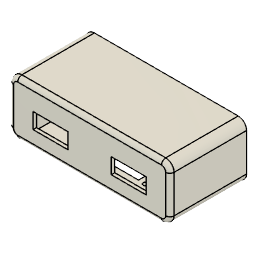
Qbot Head (Autodesk Fusion 360 design; units mm, degrees)
part number: 2026-07-07-13-50-28-448
Autodesk Fusion 360 part; units mm, degrees
sketch "Sketch1" plane through (0, 0, 0) normal (0, 0, 1) x (1, 0, 0)
  line L0 (0, 0) -> (-115, 0)
  line L1 (-115, 0) -> (-115, 39)
  line L2 (-115, 39) -> (0, 39)
  line L3 (0, 39) -> (0, 0)
  circle A0 centre (-5, 34) radius 2.6
  circle A1 centre (-5, 34) radius 1.6
  circle A2 centre (-5, 5) radius 2.6
  circle A3 centre (-5, 5) radius 1.6
  circle A4 centre (-110, 5) radius 2.6
  circle A5 centre (-110, 5) radius 1.6
  circle A6 centre (-110, 34) radius 2.6
  circle A7 centre (-110, 34) radius 1.6
  line L4 (-10, 35.5) -> (-105, 35.5)
  line L5 (-105, 35.5) -> (-105, 3.5)
  line L6 (-105, 3.5) -> (-10, 3.5)
  line L7 (-10, 3.5) -> (-10, 35.5)
  dimension "d1" = 115
  dimension "d2" = 39
  dimension "d3" = 5.2
  dimension "d4" = 5
  dimension "d5" = 5
  dimension "d6" = 3.2
  dimension "d7" = 5.2
  dimension "d8" = 5
  dimension "d9" = 5
  dimension "d10" = 3.2
  dimension "d11" = 5.2
  dimension "d12" = 5
  dimension "d13" = 5
  dimension "d14" = 3.2
  dimension "d15" = 5.2
  dimension "d16" = 5
  dimension "d17" = 5
  dimension "d18" = 3.2
  dimension "d19" = 95
  dimension "d20" = 32
  dimension "d21" = 10
  dimension "d22" = 3.5
  constraint horizontal L0
  constraint vertical L1
  constraint horizontal L2
  constraint vertical L3
  constraint coincident L0.start L3.end
  constraint concentric A0 A1
  constraint concentric A2 A3
  constraint concentric A4 A5
  constraint concentric A6 A7
  constraint horizontal L4
  constraint vertical L5
  constraint horizontal L6
  constraint vertical L7
  measures "d1" distance of L0.start L0.end
  measures "d2" distance of L0.start L2.end
  measures "d3" diameter of A0
  measures "d4" distance of L2 A0.centre
  measures "d5" distance of L3 A0.centre
  measures "d6" diameter of A1
  measures "d7" diameter of A2
  measures "d8" distance of L0 A2.centre
  measures "d9" distance of L3 A2.centre
  measures "d10" diameter of A3
  measures "d11" diameter of A4
  measures "d12" distance of L0 A4.centre
  measures "d13" distance of L1 A4.centre
  measures "d14" diameter of A5
  measures "d15" diameter of A6
  measures "d16" distance of L1 A6.centre
  measures "d17" distance of L2 A6.centre
  measures "d18" diameter of A7
  measures "d19" distance of L4.start L4.end
  measures "d20" distance of L4.start L6.end
  measures "d21" distance of L3 L7
  measures "d22" distance of L0 L6
extrude "Extrude1" add sketch "Sketch1" along normal blind 55 contours L0 L1 L2 L3 | A0 | A1 | A2 | A3 | A4 | A5 | A6 | A7 | L4 L5 L6 L7
extrude "Extrude2" cut sketch "Sketch1" along normal blind 52.5 contours L4 L5 L6 L7
extrude "Extrude3" cut sketch "Sketch1" along normal blind 5 contours A0 | A2 | A4 | A6
extrude "Extrude4" cut sketch "Sketch1" along normal blind 15 contours A1 | A3 | A5 | A7
sketch "Sketch2" plane through (0, 0, 0) normal (0, 1, 0) x (1, 0, 0)
  line L0 (-27.5, -10) -> (-82.5, -10)
  line L1 (-82.5, -10) -> (-82.5, -45)
  line L2 (-82.5, -45) -> (-27.5, -45)
  line L3 (-27.5, -45) -> (-27.5, -10)
  line L4 (-37.5, -15) -> (-72.5, -15)
  line L5 (-72.5, -15) -> (-72.5, -40)
  line L6 (-72.5, -40) -> (-37.5, -40)
  line L7 (-37.5, -40) -> (-37.5, -15)
  circle A0 centre (-32.5, -15) radius 1.6
  circle A1 centre (-32.5, -40) radius 1.6
  circle A2 centre (-77.5, -15) radius 1.6
  circle A3 centre (-77.5, -40) radius 1.6
  line L8 (0, 0) -> (-115, 0)
  line L9 (0, 0) -> (0, -55)
  dimension "d31" = 55
  dimension "d32" = 35
  dimension "d33" = 35
  dimension "d34" = 25
  dimension "d35" = 10
  dimension "d36" = 5
  dimension "d37" = 3.2
  dimension "d38" = 5
  dimension "d39" = 5
  dimension "d40" = 3.2
  dimension "d41" = 5
  dimension "d42" = 5
  dimension "d43" = 3.2
  dimension "d44" = 5
  dimension "d45" = 5
  dimension "d46" = 3.2
  dimension "d47" = 5
  dimension "d48" = 5
  dimension "d49" = 10
  dimension "d50" = 27.5
  constraint horizontal L0
  constraint vertical L1
  constraint horizontal L2
  constraint vertical L3
  constraint horizontal L4
  constraint vertical L5
  constraint horizontal L6
  constraint vertical L7
  measures "d31" distance of L0.start L0.end
  measures "d32" distance of L0.start L2.end
  measures "d33" distance of L4.start L4.end
  measures "d34" distance of L4.start L6.end
  measures "d35" distance of L3 L7
  measures "d36" distance of L0 L4
  measures "d37" diameter of A0
  measures "d38" distance of L3 A0.centre
  measures "d39" distance of L0 A0.centre
  measures "d40" diameter of A1
  measures "d41" distance of L2 A1.centre
  measures "d42" distance of L3 A1.centre
  measures "d43" diameter of A2
  measures "d44" distance of L1 A2.centre
  measures "d45" distance of L0 A2.centre
  measures "d46" diameter of A3
  measures "d47" distance of L2 A3.centre
  measures "d48" distance of L1 A3.centre
  measures "d49" distance of L0 L8
  measures "d50" distance of L3 L9
extrude "Extrude5" cut sketch "Sketch2" along normal blind 15 contours L4 L5 L6 L7
extrude "Extrude6" cut sketch "Sketch2" along normal blind 10 contours A0 | A1 | A2 | A3
ref_plane "WorkPlane1" through (0, 0, 60) normal (0, 0, 1) x (1, 0, 0)
sketch "Sketch3" plane through (0, 0, 60) normal (0, 0, 1) x (1, 0, 0)
  line L0 (-98, 23.2) -> (-73, 23.2)
  line L1 (-73, 23.2) -> (-73, 12)
  line L2 (-73, 12) -> (-98, 12)
  line L3 (-98, 12) -> (-98, 23.2)
  line L4 (-42, 23.2) -> (-17, 23.2)
  line L5 (-17, 23.2) -> (-17, 12)
  line L6 (-17, 12) -> (-42, 12)
  line L7 (-42, 12) -> (-42, 23.2)
  line L8 (0, 39) -> (-115, 39)
  line L9 (-99, 30.7) -> (-72, 30.7)
  line L10 (-72, 30.7) -> (-72, 3.7)
  line L11 (-72, 3.7) -> (-99, 3.7)
  line L12 (-99, 3.7) -> (-99, 30.7)
  line L13 (-43, 30.7) -> (-16, 30.7)
  line L14 (-16, 30.7) -> (-16, 3.7)
  line L15 (-16, 3.7) -> (-43, 3.7)
  line L16 (-43, 3.7) -> (-43, 30.7)
  line L17 (-115, 0) -> (0, 0)
  line L18 (-115, 39) -> (-115, 0)
  line L19 (0, 0) -> (0, 39)
  dimension "d56" = 25
  dimension "d57" = 11.2
  dimension "d58" = 25
  dimension "d59" = 11.2
  dimension "d61" = 27
  dimension "d62" = 27
  dimension "d63" = 7.5
  dimension "d64" = 1
  dimension "d65" = 27
  dimension "d66" = 27
  dimension "d67" = 1
  dimension "d68" = 7.5
  dimension "d69" = 3.7
  dimension "d70" = 3.7
  dimension "d73" = 16
  dimension "d74" = 16
  constraint horizontal L0
  constraint vertical L1
  constraint horizontal L2
  constraint vertical L3
  constraint horizontal L4
  constraint vertical L5
  constraint horizontal L6
  constraint vertical L7
  constraint horizontal L9
  constraint vertical L10
  constraint horizontal L11
  constraint vertical L12
  constraint horizontal L13
  constraint vertical L14
  constraint horizontal L15
  constraint vertical L16
  measures "d56" distance of L0.start L0.end
  measures "d57" distance of L0.start L2.end
  measures "d58" distance of L4.start L4.end
  measures "d59" distance of L4.start L6.end
  measures "d61" distance of L9.start L9.end
  measures "d62" distance of L9.start L11.end
  measures "d63" distance of L0 L9
  measures "d64" distance of L1 L10
  measures "d65" distance of L13.start L13.end
  measures "d66" distance of L13.start L15.end
  measures "d67" distance of L7 L16
  measures "d68" distance of L4 L13
  measures "d69" distance of L11 L17
  measures "d70" distance of L15 L17
  measures "d73" distance of L12 L18
  measures "d74" distance of L14 L19
extrude "Extrude7" cut sketch "Sketch3" against normal blind 25 contours L0 L1 L2 L3 | L4 L5 L6 L7
fillet "Fillet1" radius 6 4 edges at (0, 39, 27.5) (-115, 39, 27.5) (0, 0, 27.5) (-115, 0, 27.5)
fillet "Fillet2" radius 3 8 edges at (-113.2426, 37.2426, 55) (-115, 19.5, 55) (-113.2426, 1.7574, 55) (-57.5, 0, 55) (-1.7574, 1.7574, 55) (0, 19.5, 55) (-1.7574, 37.2426, 55) (-57.5, 39, 55)
